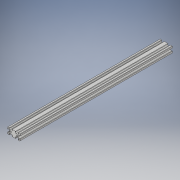
# Autodesk Inventor part: Rail_finished
Saved by Autodesk Inventor 2019 (Build 230136000, 136)
## iProperties
Created: 2021-06-18
Part Number: Rail_finished
Material: Generic
Document SubType Name: Modeling
Designer: 91742
Density: 1 g/cm^3
Appearance: Default
Author: 91742
Autodesk Inventor part; units mm, degrees
ref_plane "YZ Plane" through (0, 0, 0) normal (1, 0, 0) x (0, 1, 0)
ref_plane "XZ Plane" through (0, 0, 0) normal (0, 1, 0) x (-1, 0, 0)
ref_plane "XY Plane" through (0, 0, 0) normal (0, 0, 1) x (1, 0, 0)
sketch "Sketch1" plane through (0, 0, 0) normal (0, 0, 1) x (1, 0, 0)
  circle A0 centre (10, -0.1277) radius 2.1
  line L0 (14.5874, 9.8723) -> (19.0874, 9.8723)
  line L1 (19.0874, 9.8723) -> (14.5874, 9.8723)
  line L2 (14.5874, 9.8723) -> (13.5268, 8.8116)
  line L3 (14.5874, 9.8723) -> (16.0874, 9.8723) construction
  line L4 (13.5268, 8.8116) -> (15.9268, 8.8116)
  line L5 (6.9, -0.1277) -> (6.9, 1.7059)
  line L6 (15.9268, 6.8867) -> (13.1, 4.0599)
  line L7 (15.9268, 8.8116) -> (15.9268, 6.8867)
  line L8 (20.1068, 8.8259) -> (20.1068, 4.3259)
  line L9 (20.1068, 4.3259) -> (19.0461, 3.2652)
  line L10 (19.0461, 3.2652) -> (19.0461, 5.6652)
  line L11 (13.1, 1.8336) -> (16.9316, 5.6652)
  line L12 (19.0461, 5.6652) -> (16.9316, 5.6652)
  line L13 (13.1, 4.0599) -> (6.9, 4.0599)
  line L14 (5.4128, 10.1277) -> (0.9128, 10.1277)
  line L15 (0.9128, 10.1277) -> (5.4128, 10.1277)
  line L16 (5.4128, 10.1277) -> (3.9128, 10.1277) construction
  line L17 (4.0732, 9.0671) -> (4.0732, 6.8867)
  line L18 (5.4128, 10.1277) -> (6.4735, 9.0671)
  line L19 (4.0732, 6.8867) -> (6.9, 4.0599)
  line L20 (6.9, 1.7059) -> (3.0684, 5.5375)
  line L21 (13.1, 0) -> (13.1, 1.8336)
  line L22 (3.0684, 5.5375) -> (3.0684, 8.6839)
  line L23 (4.0732, -6.8867) -> (6.9, -4.0599)
  line L24 (6.9, -1.9614) -> (3.0684, -5.7929)
  line L25 (6.9, -0.1277) -> (6.9, -1.9614)
  line L26 (13.1, -4.0599) -> (6.9, -4.0599)
  circle A1 centre (10, -0.1277) radius 2.1
  line L27 (20.1068, -9.0813) -> (20.1068, -4.5813)
  line L28 (20.1068, -4.5813) -> (19.0461, -3.5207)
  line L29 (15.9268, -9.0671) -> (15.9268, -6.8867)
  line L30 (14.5874, -10.1277) -> (19.0874, -10.1277)
  line L31 (19.0874, -10.1277) -> (14.5874, -10.1277)
  line L32 (14.5874, -10.1277) -> (16.0874, -10.1277) construction
  line L33 (13.5268, -9.0671) -> (15.9268, -9.0671)
  line L34 (14.5874, -10.1277) -> (13.5268, -9.0671)
  line L35 (3.0684, -5.7929) -> (3.1339, -8.9387)
  line L36 (4.0732, -8.8116) -> (4.0732, -6.8867)
  line L37 (6.4732, -8.8116) -> (4.0732, -8.8116)
  line L38 (5.4126, -9.8723) -> (6.4732, -8.8116)
  line L39 (5.4126, -9.8723) -> (3.9126, -9.8723) construction
  line L40 (0.9126, -9.8723) -> (5.4126, -9.8723)
  line L41 (5.4126, -9.8723) -> (0.9126, -9.8723)
  line L42 (19.0461, -5.6652) -> (16.9316, -5.6652)
  line L43 (15.9268, -6.8867) -> (13.1, -4.0599)
  line L44 (13.1, -1.8336) -> (16.9316, -5.6652)
  line L45 (13.1, 0) -> (13.1, -1.8336)
  line L46 (19.0461, -3.5207) -> (19.0461, -5.6652)
  line L47 (-20.1068, 9.0813) -> (-20.1068, 4.5813)
  line L48 (-19.0461, 5.9207) -> (-16.9316, 5.9207)
  line L49 (-20.1068, 4.5813) -> (-19.0461, 3.5207)
  line L50 (-19.0461, 3.5207) -> (-19.0461, 5.9207)
  line L51 (-15.9277, 9.0671) -> (-15.9072, 6.9486)
  line L52 (-13.5268, 9.0671) -> (-15.9277, 9.0671)
  line L53 (-14.5874, 10.1277) -> (-19.0874, 10.1277)
  line L54 (-19.0874, 10.1277) -> (-14.5874, 10.1277)
  line L55 (-14.5874, 10.1277) -> (-16.0874, 10.1277) construction
  line L56 (-14.5874, 10.1277) -> (-13.5268, 9.0671)
  line L57 (-19.0461, -5.4098) -> (-16.9316, -5.4098)
  line L58 (-20.1068, -8.8259) -> (-20.1068, -4.3259)
  line L59 (-20.1068, -4.3259) -> (-19.0461, -3.2652)
  line L60 (-14.5874, -9.8723) -> (-19.0874, -9.8723)
  line L61 (-19.0874, -9.8723) -> (-14.5874, -9.8723)
  line L62 (-19.0461, -3.2652) -> (-19.0461, -5.4098)
  line L63 (-15.9268, -8.8116) -> (-15.9268, -6.8867)
  line L64 (-13.5268, -8.8116) -> (-15.9268, -8.8116)
  line L65 (-14.5874, -9.8723) -> (-13.5268, -8.8116)
  line L66 (-15.9268, -6.8867) -> (-13.1, -4.0599)
  line L67 (-13.1, -1.5782) -> (-16.9316, -5.4098)
  line L68 (-13.1, 0.2554) -> (-13.1, -1.5782)
  line L69 (-14.5874, -9.8723) -> (-16.0874, -9.8723) construction
  line L70 (-6.679, -2.0388) -> (-2.7685, -5.7898)
  line L71 (-4.0732, -6.8867) -> (-6.9, -4.0599)
  line L72 (-6.4732, -8.8116) -> (-4.0732, -8.8116)
  line L73 (-5.4126, -9.8723) -> (-6.4732, -8.8116)
  line L74 (-4.0732, -8.8116) -> (-4.0732, -6.8867)
  line L75 (-2.7685, -5.7898) -> (-2.7031, -8.9355)
  line L76 (-5.4126, -9.8723) -> (-3.9126, -9.8723) construction
  line L77 (-0.9126, -9.8723) -> (-5.4126, -9.8723)
  line L78 (-5.4126, -9.8723) -> (-0.9126, -9.8723)
  line L79 (-0.5477, -8.8907) -> (0.6007, -8.8668)
  line L80 (-2.7031, -8.9355) -> (-0.5477, -8.8907)
  line L81 (-6.7171, -0.2055) -> (-6.7553, 1.6277)
  line L82 (-5.4124, 10.1277) -> (-0.9124, 10.1277)
  line L83 (-0.9124, 10.1277) -> (-5.4124, 10.1277)
  line L84 (-5.4124, 10.1277) -> (-3.9124, 10.1277) construction
  line L85 (-4.0736, 9.0671) -> (-4.0542, 7.0634)
  line L86 (-6.473, 9.0671) -> (-4.0736, 9.0671)
  line L87 (-5.4124, 10.1277) -> (-6.473, 9.0671)
  line L88 (-4.0542, 7.0634) -> (-6.8535, 4.2094)
  line L89 (-6.7553, 1.6277) -> (-3.0043, 5.5382)
  line L90 (-3.0043, 5.5382) -> (-3.0698, 8.6839)
  line L91 (-0.9124, 10.1277) -> (0.2363, 10.1277)
  circle A2 centre (-10, 0.1277) radius 2.1
  line L92 (-15.9072, 6.9486) -> (-13.0532, 4.1494)
  line L93 (-13.1, 2.0891) -> (-16.9316, 5.9207)
  line L94 (-13.1, 0.2554) -> (-13.1, 2.0891)
  circle A3 centre (-10, 0.1277) radius 2.1
  line L95 (-13.1, -4.0599) -> (-6.9, -4.0599)
  line L96 (-6.7171, -0.2055) -> (-6.679, -2.0388)
  line L97 (-13.0532, 4.1494) -> (-6.8535, 4.2094)
  line L98 (-20.1068, 9.0813) -> (-20.1068, 9.1277)
  line L99 (-19.1068, 10.1277) -> (-19.0874, 10.1277)
  arc A4 (-19.1068, 10.1277) -> (-20.1068, 9.1277) centre (-19.1068, 9.1277) ccw
  line L100 (19.0874, 9.8723) -> (19.1068, 9.8723)
  line L101 (20.1068, 8.8723) -> (20.1068, 8.8259)
  arc A5 (20.1068, 8.8723) -> (19.1068, 9.8723) centre (19.1068, 8.8723) ccw
  line L102 (19.0874, -10.1277) -> (19.1068, -10.1277)
  line L103 (20.1068, -9.1277) -> (20.1068, -9.0671)
  arc A6 (19.1068, -10.1277) -> (20.1068, -9.1277) centre (19.1068, -9.1277) ccw
  line L104 (-20.1068, -8.8259) -> (-20.1068, -8.8723)
  line L105 (-19.1068, -9.8723) -> (-19.0874, -9.8723)
  arc A7 (-20.1068, -8.8723) -> (-19.1068, -9.8723) centre (-19.1068, -8.8723) ccw
  line L106 (-15.9268, -8.8116) -> (-13.5268, -8.8116)
  line L107 (-14.5874, -9.8723) -> (-19.1068, -9.8723)
  line L108 (-20.1068, -8.8723) -> (-20.1068, -4.3259)
  line L109 (-19.0461, -3.2652) -> (-19.0461, -5.4098)
  line L110 (-16.9316, -5.4098) -> (-13.1, -1.5782)
  line L111 (-13.1, 2.0891) -> (-16.9316, 5.9207)
  line L112 (-19.0461, 5.9207) -> (-19.0461, 3.5207)
  line L113 (-20.1068, 4.5813) -> (-20.1068, 9.0959)
  line L114 (-19.1068, 10.1277) -> (-14.5874, 10.1277)
  line L115 (-13.5268, 9.0671) -> (-15.9277, 9.0671)
  line L116 (-15.9072, 6.9486) -> (-13.0532, 4.1494)
  line L117 (-6.8535, 4.2094) -> (-4.0542, 7.0634)
  line L118 (-4.0736, 9.0671) -> (-6.473, 9.0671)
  line L119 (-5.4124, 10.1277) -> (5.4128, 10.1277)
  line L120 (4.0732, 6.8867) -> (6.9, 4.0599)
  line L121 (13.1, 4.0599) -> (15.9268, 6.8867)
  line L122 (15.9268, 8.8116) -> (13.5268, 8.8116)
  line L123 (14.5874, 9.8723) -> (19.1068, 9.8723)
  line L124 (-0.9126, -9.8723) -> (0.9126, -9.8723)
  line L125 (4.0732, 9.0671) -> (6.4735, 9.0671)
  line L126 (-2.7031, -8.9355) -> (3.1313, -8.8141)
  line L127 (-3.0698, 8.6839) -> (3.0684, 8.6839)
  point P0 (0, 0)
  point P1 (-20.1068, 10.1277)
  point P2 (20.1068, 9.8723)
  point P3 (20.1068, -10.1277)
  point P4 (-20.1068, -9.8723)
  dimension "d42" = 4.2
  dimension "d43" = 4.5
  dimension "d44" = 1.5
  dimension "d45" = 135
  dimension "d46" = 2.4
  dimension "d47" = 3.1
  dimension "d48" = 4.5
  dimension "d49" = 1.5
  dimension "d50" = 2.4
  dimension "d51" = 6.2
  dimension "d52" = 1
  dimension "d53" = 1
  dimension "d54" = 1
  dimension "d55" = 1
  dimension "d58" = 10
  dimension "d59" = 10
  dimension "d60" = 10
  dimension "d61" = 10
  dimension "d62" = 20
  constraints: 256 end point, 17 point on line, 14 collinear, 10 point on circle, 8 centre point, 8 tangent, 7 perpendicular, 6 horizontal, 6 vertical, 1 equal length, 1 parallel
  measures "d42" diameter of A0
  measures "d43" distance of L0.start L0.end
  measures "d44" distance of L0.start L4.start
  measures "d45" angle of L2 L3
  measures "d46" distance of L4.start L7.start
  measures "d47" distance of A0.centre L5.start
  measures "d48" distance of L101.end L8.end
  measures "d49" distance of L8.end L10.start
  measures "d50" distance of L10.start L12.start
  measures "d51" distance of L13.end L6.end
  measures "d52" radius of A4
  measures "d53" radius of A5
  measures "d54" radius of A6
  measures "d55" radius of A7
  measures "d58" distance from line of L30 A0.centre
  measures "d59" distance from line of L60 A2.centre
  measures "d60" distance from line of L53 A2.centre
  measures "d61" distance from line of L0 A0.centre
  measures "d62" horizontal distance of A2.centre A0.centre
extrude "Extrusion1" add sketch "Sketch1" along normal blind 490 contours L0 L100 A5 L101 L8 L9 L10 L12 L11 L21 L45 L44 L42 L46 L28 L27 L103 A6 L102 L30 L34 L33 L29 L43 L26 L23 L36 L37 L38 L40 L124 L77 L73 L72 L74 L71 L95 L66 L63 L64 L65 L60 L105 A7 L104 L58 L59 L62 L57 L67 L68 L94 L93 L48 L50 L49 L47 L98 A4 L99 L53 L56 L52 L51 L92 L97 L88 L85 L86 L87 L82 L91 L119 L14 L18 L125 L17 L19 L13 L6 L7 L4 L2 | L25 L24 L35 L126 L79 L80 L75 L70 L96 L81 L89 L90 L127 L22 L20 L5
body "Solid1"
